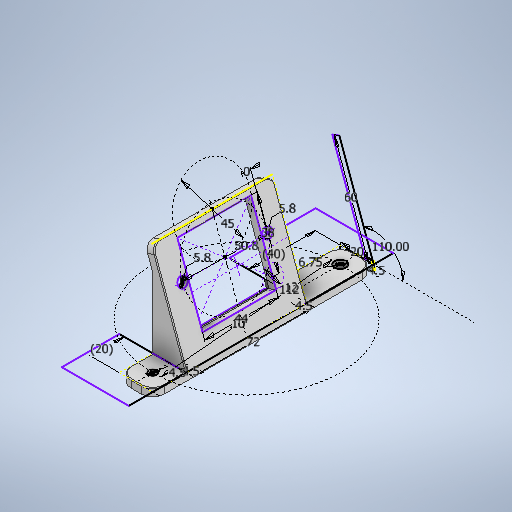
# Autodesk Inventor part: ThriftyCamMountTopSwerve2
Saved by Autodesk Inventor 2025 (Build 290162000, 162)
## iProperties
Created: 2025-03-15
Part Number: ThriftyCamMountTopSwerve2
Material: Generic
Document SubType Name: Modeling
Designer: john
Density: 1 g/cm^3
Appearance: Default
Author: john
Autodesk Inventor part; units mm, degrees
ref_plane "YZ Plane" through (0, 0, 0) normal (1, 0, 0) x (0, 1, 0)
ref_plane "XZ Plane" through (0, 0, 0) normal (0, 1, 0) x (-1, 0, 0)
ref_plane "XY Plane" through (0, 0, 0) normal (0, 0, 1) x (1, 0, 0)
sketch "Sketch1" plane through (0, 0, 0) normal (0, 0, 1) x (1, 0, 0)
  line L0 (-10, -2.25) -> (10, -2.25)
  line L1 (10, -2.25) -> (10, 2.25)
  line L2 (10, 2.25) -> (-10, 2.25)
  line L3 (-10, 2.25) -> (-10, -2.25)
  line L4 (-10, -2.25) -> (10, 2.25) construction
  line L5 (10, -2.25) -> (-10, 2.25) construction
  line L6 (10, 2.25) -> (-10.5212, 58.6316)
  line L7 (10, 2.25) -> (70, 2.25) construction
  line L8 (-10.5212, 58.6316) -> (-14.7498, 57.0925)
  line L9 (5.2112, 2.25) -> (-14.7498, 57.0925)
  point P0 (0, 0)
  dimension "d0" = 20
  dimension "d1" = 4.5
  dimension "d11" = 60
  dimension "d12" = 110
  constraints: 20 end point, 3 parallel, 2 horizontal, 2 midpoint, 1 equal length, 1 perpendicular, 1 point on line
  measures "d0" distance of L2.end L1.end
  measures "d1" distance of L1.end L0.end
  measures "d11" distance of L1.end L6.end
  measures "d12" angle of L7 L6
extrude "Extrusion1" add sketch "Sketch1" along normal blind 132 contours L3 L2 L1 L0
sketch "Sketch2" plane through (-10, 2.25, 0) normal (0, 1, 0) x (1, 0, 0)
  line L0 (20, -132) -> (0, -132) construction
  line L1 (10, -132) -> (10, 0) construction
  line L2 (20, 0) -> (0, 0) construction
  line L3 (0, 0) -> (0, -132) construction
  line L4 (0, -66) -> (20, -66) construction
  line L5 (20, 0) -> (20, -132) construction
  circle A0 centre (10, -66) radius 56 construction
  circle A1 centre (10, -122) radius 2.25
  circle A2 centre (10, -10) radius 3.375
  line L6 (0, -76) -> (20, -76) construction
  line L7 (0, -112) -> (20, -112)
  line L8 (20, -112) -> (20, -40)
  line L9 (20, -40) -> (0, -40)
  line L10 (0, -40) -> (0, -112)
  line L11 (0, -112) -> (20, -40) construction
  line L12 (20, -112) -> (0, -40) construction
  line L13 (20, -112) -> (-19.9682, -112)
  line L14 (-19.9682, -112) -> (-19.9682, -146.3538)
  line L15 (-19.9682, -146.3538) -> (20, -146.3538)
  line L16 (20, -146.3538) -> (20, -112)
  line L17 (20, -40) -> (-26.4005, -40)
  line L18 (-26.4005, -40) -> (-26.4005, 11.7001)
  line L19 (-26.4005, 11.7001) -> (20, 11.7001)
  line L20 (20, 11.7001) -> (20, -40)
  line L21 (0, -40) -> (15.0422, -40)
  line L22 (15.0422, -40) -> (15.0422, -44.5)
  line L23 (15.0422, -44.5) -> (0, -44.5)
  line L24 (0, -44.5) -> (0, -40)
  line L25 (0, -107.5) -> (15.0422, -107.5)
  line L26 (15.0422, -107.5) -> (15.0422, -112)
  line L27 (15.0422, -112) -> (0, -112)
  line L28 (0, -112) -> (0, -107.5)
  point P0 (10, -76)
  point P1 (0, -40)
  point P2 (20, -112)
  point P3 (0, -112)
  point P4 (0, -107.5)
  point P5 (0, -44.5)
  dimension "d4" = 112
  dimension "d5" = 4.5
  dimension "d6" = 6.75
  dimension "d9" = 10
  dimension "d10" = 72
  dimension "d16" = 20
  dimension "d17" = 40
  dimension "d36" = 4.5
  dimension "d37" = 4.5
  constraints: 50 end point, 11 parallel, 7 midpoint, 6 perpendicular, 5 horizontal, 4 coincident, 3 centre point, 3 point on line, 2 point on circle
  measures "d4" diameter of A0
  measures "d5" diameter of A1
  measures "d6" diameter of A2
  measures "d9" distance between parallel lines of L4 L6
  measures "d10" distance of L8.end L7.end
  measures "d16" distance between parallel lines of L0 L7
  measures "d17" distance between parallel lines of L2 L9
  measures "d36" distance of L21.end L22.end
  measures "d37" distance of L26.start L27.start
extrude "Extrusion2" cut sketch "Sketch2" against normal blind 132 contours A1 | A2
extrude "Extrusion3" add sketch "Sketch1" along normal blind 132 contours L2 L9 L8 L6
sketch "Sketch3" plane through (10, -2.25, 132) normal (1, 0, 0) x (0, 0, -1)
  point P0 (132, 2.25)
extrude "Extrusion4" cut sketch "Sketch2" along normal blind 132 contours A1 | A2 | L7 L16 L15 L14 L13 | L9 L17 L18 L19 L20
sketch "Sketch4" plane through (-10.5212, 58.6316, 112) normal (0.9396926, 0.3420201, 0) x (0, 0, -1)
  line L0 (72, 0) -> (0, 0) projected
  line L1 (36, 0) -> (36, -57.7119) construction
  line L2 (72, 0) -> (72, -58.3621) construction
  line L3 (72, -28.8559) -> (10, -28.8559) construction
  circle A0 centre (36, 0) radius 22.5 construction
  line L4 (67, -22.5) -> (5, -22.5) construction
  circle A1 centre (36, -22.5) radius 25.4 construction
  circle A2 centre (10.6, -22.5) radius 2.9
  circle A3 centre (61.4, -22.5) radius 2.9
  line L5 (14, -3.5) -> (58, -3.5)
  line L6 (58, -3.5) -> (58, -41.5)
  line L7 (58, -47.5) -> (14, -47.5)
  line L8 (14, -47.5) -> (14, -3.5)
  line L9 (14, -3.5) -> (58, -41.5) construction
  line L10 (58, -3.5) -> (14, -41.5) construction
  circle A4 centre (58, -41.5) radius 6 construction
  line L11 (58, -47.5) -> (58, -41.5)
  point P0 (112, -58.6941)
  point P1 (41, -28.8559)
  dimension "d20" = 45
  dimension "d28" = 12
  dimension "d21" = 50.8
  dimension "d22" = 5.8
  dimension "d23" = 5.8
  dimension "d26" = 44
  dimension "d27" = 38
  dimension "d35" = 0
  constraints: 20 end point, 4 midpoint, 4 point on line, 3 centre point, 3 coincident, 3 horizontal, 3 point on circle, 2 parallel, 2 perpendicular, 2 vertical alignment, 1 vertical, 4 other
  measures "d21" diameter of A1
  measures "d22" diameter of A2
  measures "d23" diameter of A3
  measures "d26" distance of L7.end L7.start
  measures "d27" distance of L6.end L5.end
  measures "d35" distance of point (61.4, -22.5) A3.centre
extrude "Extrusion5" cut sketch "Sketch4" against normal blind 12 contours A2 | A3
extrude "Extrusion6" cut sketch "Sketch4" against normal blind 6 contours L5 L6 L11 L7 L8
fillet "Fillet1" radius 3 1 edges at (5.2112, 2.25, 76)
fillet "Fillet2" radius 7 4 edges at (10, 0, 132) (-10, 0, 132) (-10, 0, 0) (10, 0, 0)
fillet "Fillet3" radius 5 2 edges at (-12.6355, 57.862, 40) (-12.6355, 57.862, 112)
fillet "Fillet4" radius 0.5 14 edges at (-10.0203, 57.2554, 110.5355) (-10.5212, 58.6316, 76) (-10.0203, 57.2554, 41.4645) (0.5944, 28.0915, 40) (0.5944, 28.0915, 112) (7.9497, 2.25, 2.0503) (0, 2.25, 0) (-7.9497, 2.25, 2.0503) (-10, 2.25, 66) (-7.9497, 2.25, 129.9497) (0, 2.25, 132) (7.9497, 2.25, 129.9497) (10, 2.25, 118.5) (10, 2.25, 23.5)
sketch "Sketch5" plane through (0.9268, 2.25, 112) normal (0, 1, 0) x (1, 0, 0)
  point P0 (-0.9268, 112)
extrude "Extrusion7" add sketch "Sketch2" along normal up to surface contours L10 L25 L26 L7 | L10 L9 L22 L23 surface through (-14.7498, 57.0925, 0) normal (-0.9396926, -0.3420201, 0)
body "Solid1"
